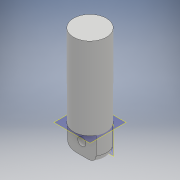
# Autodesk Inventor part: CosaCuello
Saved by Autodesk Inventor 2017 SP1 (Build 210196100, 196)
## iProperties
Part Number: CosaCuello
Material: Genérico
Document SubType Name: Modeling
Designer: Juan
Density: 1 g/cm^3
Appearance: Valor por defecto
Author: Juan
Autodesk Inventor part; units mm, degrees
ref_plane "YZ Plane" through (0, 0, 0) normal (1, 0, 0) x (0, 1, 0)
ref_plane "XZ Plane" through (0, 0, 0) normal (0, 1, 0) x (-1, 0, 0)
ref_plane "XY Plane" through (0, 0, 0) normal (0, 0, 1) x (1, 0, 0)
sketch "Boceto1" plane through (0, 0, 0) normal (1, 0, 0) x (0, 1, 0)
  line L0 (5.2272, 23.4487) -> (5.2272, -26.5513)
  line L1 (15.2272, -26.5513) -> (15.2272, 23.4487)
  line L2 (5.2272, -26.5513) -> (15.2272, -26.5513)
  line L3 (5.2272, 23.4487) -> (15.2272, 23.4487)
  point P0 (0, 0)
  dimension "d0" = 10
  dimension "d1" = 50
  dimension "d2" = 50
  constraints: 8 end point, 1 horizontal, 1 vertical
  measures "d0" distance of L1.end L0.start
  measures "d1" distance of L0.start L0.end
  measures "d2" distance of L1.start L1.end
revolve "Revolución1" add sketch "Boceto1" angle 360 about axis through (0, 5.2272, 23.4487) along (0, 0, -1)
ref_plane "Plano de trabajo1" through (0, 5.2272, -26.5513) normal (0, 0, -1) x (-1, 0, 0)
sketch "Boceto2" plane through (0, 5.2272, -26.5513) normal (0, 0, -1) x (-1, 0, 0)
  line L0 (8.6603, -5) -> (-8.6603, -5)
  line L1 (8.6603, 5) -> (-8.6603, 5)
  arc A0 (8.6603, -5) -> (8.6603, 5) centre (0, 0) ccw
  arc A1 (-8.6603, 5) -> (-8.6603, -5) centre (0, 0) ccw
  point P0 (0, -5.2272)
  point P1 (0, 0)
  dimension "d32" = 10
  dimension "d33" = 10
  dimension "d34" = 10
  dimension "d35" = 5
  dimension "d36" = 5
  dimension "d37" = 5
  dimension "d38" = 10
  dimension "d39" = 0
  constraints: 4 end point, 4 point on circle, 2 centre point, 1 horizontal, 1 parallel
  measures "d32" radius of A0
  measures "d33" radius of A1
  measures "d34" distance between parallel lines of L0 L1
  measures "d35" distance from line of point (0, 0) L1
  measures "d36" distance from line of A0.centre L1
  measures "d37" distance from line of A1.centre L1
  measures "d38" distance of point (0, 0) L1.start
  measures "d39" distance of point (0, 0) A1.centre
extrude "Extrusión1" add sketch "Boceto2" along normal blind 15
sketch "Boceto5" plane through (0, 5.2272, -26.5513) normal (0, 0, -1) x (-1, 0, 0)
  point P0 (0, -5.2272)
ref_plane "Plano de trabajo4" through (-8.6603, 10.2272, -26.5513) normal (0, 1, 0) x (1, 0, 0)
sketch "Boceto6" plane through (-8.6603, 10.2272, -26.5513) normal (0, 1, 0) x (1, 0, 0)
  line L0 (0, 15) -> (-1.3397, 15) construction
  line L1 (17.3205, 0) -> (0, 0) construction
  line L2 (0, 15) -> (17.3205, 0) construction
  line L3 (17.3205, 15) -> (0, 0) construction
  point P0 (8.6603, -26.5513)
  constraints: 4 end point
hole "Agujero3" at (-0.0048, 10.2272, -34.0496) direction (0, -1, 0) diameter 5 end through all
fillet "Empalme1" radius 4 2 edges at (10, 5.2272, -41.5513) (-10, 5.2272, -41.5513)
